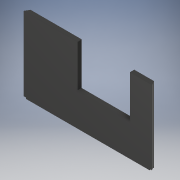
# Autodesk Inventor part: BA03
Saved by Autodesk Inventor 2017 (Build 210142000, 142)
## iProperties
Created: 2018-10-18
Part Number: BA03
Material: ABS Plastic
Document SubType Name: Modeling
Designer: Dell
Density: 1.06 g/cm^3
Appearance: Smooth - Black
Author: Dell
Autodesk Inventor part; units mm, degrees
ref_plane "YZ Plane" through (0, 0, 0) normal (1, 0, 0) x (0, 1, 0)
ref_plane "XZ Plane" through (0, 0, 0) normal (0, 1, 0) x (-1, 0, 0)
ref_plane "XY Plane" through (0, 0, 0) normal (0, 0, 1) x (1, 0, 0)
sketch "Sketch1" plane through (0, 0, 0) normal (0, 0, 1) x (1, 0, 0)
  line L0 (0, 0) -> (292.1, 0)
  line L1 (292.1, 0) -> (292.1, -177.8)
  line L2 (292.1, -177.8) -> (0, -177.8)
  line L3 (0, -177.8) -> (0, 0)
  dimension "d0" = 292.1
  dimension "d1" = 177.8
  constraints: 8 end point, 2 parallel, 1 horizontal, 1 perpendicular
  measures "d0" distance of L1.end L2.end
  measures "d1" distance of L0.end L1.end
extrude "Extrusion1" add sketch "Sketch1" along normal blind 10
sketch "Sketch2" plane through (0, 0, 0) normal (0, 1, 0) x (1, 0, 0)
  line L0 (292.1, -10) -> (0, -10) projected
  line L1 (0, -10) -> (-5.7735, -10)
  line L2 (-5.7735, -10) -> (0, 0)
  line L3 (0, 0) -> (0, -10) projected
  line L4 (0, 0) -> (0, -10) projected
  line L5 (0, -10) -> (0, 0)
  line L6 (292.1, -10) -> (297.8735, -10)
  line L7 (292.1, 0) -> (292.1, -10) projected
  line L8 (297.8735, -10) -> (292.1, 0)
  line L9 (292.1, 0) -> (292.1, -10)
  dimension "d4" = 30
  dimension "d5" = 60
  constraints: 12 end point, 2 collinear, 2 horizontal
  measures "d4" angle of L3 L2
  measures "d5" angle of L6 L8
extrude "Extrusion2" add sketch "Sketch2" against normal blind 175
sketch "Sketch3" plane through (0, 0, 10) normal (0, 0, 1) x (1, 0, 0)
  line L0 (46.05, -100) -> (246.05, -100)
  line L1 (246.05, -100) -> (246.05, 0)
  line L2 (246.05, 0) -> (46.05, 0)
  line L3 (46.05, 0) -> (46.05, -100)
  line L4 (-5.7735, 0) -> (297.8735, 0) projected
  line L5 (46.05, -100) -> (121.05, -100)
  line L6 (121.05, -100) -> (121.05, 0)
  line L7 (121.05, 0) -> (46.05, 0)
  line L8 (46.05, 0) -> (46.05, -100)
  point P0 (0, 0)
  point P1 (146.05, 0)
  dimension "d8" = 200
  dimension "d9" = 100
  dimension "d12" = 75
  constraints: 16 end point, 4 parallel, 2 horizontal, 2 midpoint, 2 perpendicular, 1 point on line
  measures "d8" distance of L1.end L2.end
  measures "d9" distance of L0.end L1.end
  measures "d12" distance between parallel lines of L3 L6
extrude "Extrusion3" cut sketch "Sketch3" against normal through all contours L6 L2 L1 L0
body "Solid1"
